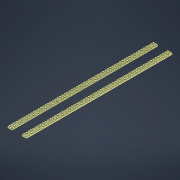
# Autodesk Inventor part: 110033226_ipt_39_背流基座
Saved by Autodesk Inventor 2022 (Build 260153000, 153)
## iProperties
Created: 2022-06-26
Part Number: 110033226_ipt_39_背流基座
Material: 一般
Document SubType Name: Modeling
Designer: User
Density: 1 g/cm^3
Appearance: 預設
Author: User
Autodesk Inventor part; units mm, degrees
ref_plane "YZ Plane" through (0, 0, 0) normal (1, 0, 0) x (0, 1, 0)
ref_plane "XZ Plane" through (0, 0, 0) normal (0, 1, 0) x (-1, 0, 0)
ref_plane "XY Plane" through (0, 0, 0) normal (0, 0, 1) x (1, 0, 0)
sketch "草圖1" plane through (0, 0, 0) normal (0, 1, 0) x (-1, 0, 0)
  line L0 (0, 0) -> (40, 0)
  line L1 (40, 0) -> (40, -305)
  line L2 (40, -305) -> (0, -305)
  line L3 (0, -305) -> (0, 0)
  circle A0 centre (2.5, -2.5) radius 1.7
  line L4 (10, -305) -> (10, 0)
  line L5 (30, -305) -> (30, 0)
  dimension "d0" = 40
  dimension "d1" = 305
  dimension "d2" = 3.4
  dimension "d3" = 2.5
  dimension "d4" = 2.5
  dimension "d45" = 10
  dimension "d46" = 10
  constraints: 12 end point, 4 point on line, 3 perpendicular, 2 parallel, 1 centre point, 1 horizontal
  measures "d0" distance of L1.end L2.end
  measures "d1" distance of L0.end L1.end
  measures "d2" diameter of A0
  measures "d3" distance from line of L3 A0.centre
  measures "d4" distance from line of L0 A0.centre
  measures "d45" distance between parallel lines of L3 L4
  measures "d46" distance between parallel lines of L1 L5
extrude "擠出1" add sketch "草圖1" along normal blind 2.5 contours L0 L4 L2 L3 | L0 L1 L2 L5 | A0
extrude "擠出2" cut sketch "草圖1" along normal blind 1.5 contours A0
sketch "草圖2" plane through (0, 2.5, 0) normal (0, 1, 0) x (1, 0, 0)
  circle A0 centre (-2.5, 2.5) radius 1.7 projected
  point P0 (0, 0)
extrude "擠出3" add sketch "草圖2" along normal blind 1.5
pattern_linear "矩形陣列3" count 61 spacing 5 along (0, 0, -1) count 2 spacing 5 along (-1, 0, 0) of "擠出3", "擠出2"
sketch "草圖3" plane through (0, 2.5, 0) normal (0, 1, 0) x (1, 0, 0)
  circle A0 centre (-2.5, 2.5) radius 1.7 projected
  line L0 (0, 305) -> (0, 0) projected
  line L1 (-30, 0) -> (-40, 0) projected
  line L2 (-40, 0) -> (-40, 305) projected
  line L3 (-40, 305) -> (-30, 305) projected
  circle A1 centre (-2.5, 7.5) radius 1.7 projected
  circle A2 centre (-2.5, 12.5) radius 1.7 projected
  circle A3 centre (-2.5, 17.5) radius 1.7 projected
  circle A4 centre (-2.5, 22.5) radius 1.7 projected
  circle A5 centre (-2.5, 27.5) radius 1.7 projected
  circle A6 centre (-2.5, 32.5) radius 1.7 projected
  circle A7 centre (-2.5, 37.5) radius 1.7 projected
  circle A8 centre (-2.5, 42.5) radius 1.7 projected
  circle A9 centre (-2.5, 47.5) radius 1.7 projected
  circle A10 centre (-2.5, 52.5) radius 1.7 projected
  circle A11 centre (-2.5, 57.5) radius 1.7 projected
  circle A12 centre (-2.5, 62.5) radius 1.7 projected
  circle A13 centre (-2.5, 67.5) radius 1.7 projected
  circle A14 centre (-2.5, 72.5) radius 1.7 projected
  circle A15 centre (-2.5, 77.5) radius 1.7 projected
  circle A16 centre (-2.5, 82.5) radius 1.7 projected
  circle A17 centre (-2.5, 87.5) radius 1.7 projected
  circle A18 centre (-2.5, 92.5) radius 1.7 projected
  circle A19 centre (-2.5, 97.5) radius 1.7 projected
  circle A20 centre (-2.5, 102.5) radius 1.7 projected
  circle A21 centre (-2.5, 107.5) radius 1.7 projected
  circle A22 centre (-2.5, 112.5) radius 1.7 projected
  circle A23 centre (-2.5, 117.5) radius 1.7 projected
  circle A24 centre (-2.5, 122.5) radius 1.7 projected
  circle A25 centre (-2.5, 127.5) radius 1.7 projected
  circle A26 centre (-2.5, 132.5) radius 1.7 projected
  circle A27 centre (-2.5, 137.5) radius 1.7 projected
  circle A28 centre (-2.5, 142.5) radius 1.7 projected
  circle A29 centre (-2.5, 147.5) radius 1.7 projected
  circle A30 centre (-2.5, 152.5) radius 1.7 projected
  circle A31 centre (-2.5, 157.5) radius 1.7 projected
  circle A32 centre (-2.5, 162.5) radius 1.7 projected
  circle A33 centre (-2.5, 167.5) radius 1.7 projected
  circle A34 centre (-2.5, 172.5) radius 1.7 projected
  circle A35 centre (-2.5, 177.5) radius 1.7 projected
  circle A36 centre (-2.5, 182.5) radius 1.7 projected
  circle A37 centre (-2.5, 187.5) radius 1.7 projected
  circle A38 centre (-2.5, 192.5) radius 1.7 projected
  circle A39 centre (-2.5, 197.5) radius 1.7 projected
  circle A40 centre (-2.5, 202.5) radius 1.7 projected
  circle A41 centre (-2.5, 207.5) radius 1.7 projected
  circle A42 centre (-2.5, 212.5) radius 1.7 projected
  circle A43 centre (-2.5, 217.5) radius 1.7 projected
  circle A44 centre (-2.5, 222.5) radius 1.7 projected
  circle A45 centre (-2.5, 227.5) radius 1.7 projected
  circle A46 centre (-2.5, 232.5) radius 1.7 projected
  circle A47 centre (-2.5, 237.5) radius 1.7 projected
  circle A48 centre (-2.5, 242.5) radius 1.7 projected
  circle A49 centre (-2.5, 247.5) radius 1.7 projected
  circle A50 centre (-2.5, 252.5) radius 1.7 projected
  circle A51 centre (-2.5, 257.5) radius 1.7 projected
  circle A52 centre (-2.5, 262.5) radius 1.7 projected
  circle A53 centre (-2.5, 267.5) radius 1.7 projected
  circle A54 centre (-2.5, 272.5) radius 1.7 projected
  circle A55 centre (-2.5, 277.5) radius 1.7 projected
  circle A56 centre (-2.5, 282.5) radius 1.7 projected
  circle A57 centre (-2.5, 287.5) radius 1.7 projected
  circle A58 centre (-2.5, 292.5) radius 1.7 projected
  circle A59 centre (-2.5, 297.5) radius 1.7 projected
  circle A60 centre (-2.5, 302.5) radius 1.7 projected
  circle A61 centre (-7.5, 2.5) radius 1.7 projected
  circle A62 centre (-7.5, 7.5) radius 1.7 projected
  circle A63 centre (-7.5, 12.5) radius 1.7 projected
  circle A64 centre (-7.5, 17.5) radius 1.7 projected
  circle A65 centre (-7.5, 22.5) radius 1.7 projected
  circle A66 centre (-7.5, 27.5) radius 1.7 projected
  circle A67 centre (-7.5, 32.5) radius 1.7 projected
  circle A68 centre (-7.5, 37.5) radius 1.7 projected
  circle A69 centre (-7.5, 42.5) radius 1.7 projected
  circle A70 centre (-7.5, 47.5) radius 1.7 projected
  circle A71 centre (-7.5, 52.5) radius 1.7 projected
  circle A72 centre (-7.5, 57.5) radius 1.7 projected
  circle A73 centre (-7.5, 62.5) radius 1.7 projected
  circle A74 centre (-7.5, 67.5) radius 1.7 projected
  circle A75 centre (-7.5, 72.5) radius 1.7 projected
  circle A76 centre (-7.5, 77.5) radius 1.7 projected
  circle A77 centre (-7.5, 82.5) radius 1.7 projected
  circle A78 centre (-7.5, 87.5) radius 1.7 projected
  circle A79 centre (-7.5, 92.5) radius 1.7 projected
  circle A80 centre (-7.5, 97.5) radius 1.7 projected
  circle A81 centre (-7.5, 102.5) radius 1.7 projected
  circle A82 centre (-7.5, 107.5) radius 1.7 projected
  circle A83 centre (-7.5, 112.5) radius 1.7 projected
  circle A84 centre (-7.5, 117.5) radius 1.7 projected
  circle A85 centre (-7.5, 122.5) radius 1.7 projected
  circle A86 centre (-7.5, 127.5) radius 1.7 projected
  circle A87 centre (-7.5, 132.5) radius 1.7 projected
  circle A88 centre (-7.5, 137.5) radius 1.7 projected
  circle A89 centre (-7.5, 142.5) radius 1.7 projected
  circle A90 centre (-7.5, 147.5) radius 1.7 projected
  circle A91 centre (-7.5, 152.5) radius 1.7 projected
  circle A92 centre (-7.5, 157.5) radius 1.7 projected
  circle A93 centre (-7.5, 162.5) radius 1.7 projected
  circle A94 centre (-7.5, 167.5) radius 1.7 projected
  circle A95 centre (-7.5, 172.5) radius 1.7 projected
  circle A96 centre (-7.5, 177.5) radius 1.7 projected
  circle A97 centre (-7.5, 182.5) radius 1.7 projected
  circle A98 centre (-7.5, 187.5) radius 1.7 projected
  circle A99 centre (-7.5, 192.5) radius 1.7 projected
  circle A100 centre (-7.5, 197.5) radius 1.7 projected
  circle A101 centre (-7.5, 202.5) radius 1.7 projected
  circle A102 centre (-7.5, 207.5) radius 1.7 projected
  circle A103 centre (-7.5, 212.5) radius 1.7 projected
  circle A104 centre (-7.5, 217.5) radius 1.7 projected
  circle A105 centre (-7.5, 222.5) radius 1.7 projected
  circle A106 centre (-7.5, 227.5) radius 1.7 projected
  circle A107 centre (-7.5, 232.5) radius 1.7 projected
  circle A108 centre (-7.5, 237.5) radius 1.7 projected
  circle A109 centre (-7.5, 242.5) radius 1.7 projected
  circle A110 centre (-7.5, 247.5) radius 1.7 projected
  circle A111 centre (-7.5, 252.5) radius 1.7 projected
  circle A112 centre (-7.5, 257.5) radius 1.7 projected
  circle A113 centre (-7.5, 262.5) radius 1.7 projected
  circle A114 centre (-7.5, 267.5) radius 1.7 projected
  circle A115 centre (-7.5, 272.5) radius 1.7 projected
  circle A116 centre (-7.5, 277.5) radius 1.7 projected
  circle A117 centre (-7.5, 282.5) radius 1.7 projected
  circle A118 centre (-7.5, 287.5) radius 1.7 projected
  circle A119 centre (-7.5, 292.5) radius 1.7 projected
  circle A120 centre (-7.5, 297.5) radius 1.7 projected
  circle A121 centre (-7.5, 302.5) radius 1.7 projected
  circle A122 centre (-37.5, 2.5) radius 1.7
  line L4 (-30, 305) -> (-30, 0) projected
  line L5 (0, 0) -> (-10, 0) projected
  line L6 (-10, 0) -> (-10, 305) projected
  line L7 (-10, 305) -> (0, 305) projected
  dimension "d26" = 3.4
  dimension "d27" = 2.5
  dimension "d28" = 2.5
  constraints: 1 centre point
  measures "d26" diameter of A122
  measures "d27" distance from line of L2 A122.centre
  measures "d28" distance from line of L1 A122.centre
extrude "擠出4" add sketch "草圖3" along normal blind 1.5 contours A122
pattern_linear "矩形陣列4" count 61 spacing 5 along (0, 0, -1) count 2 spacing 5 along (1, 0, 0) of "擠出4"
sketch "草圖4" plane through (0, 0, 0) normal (0, -1, 0) x (1, 0, 0)
  circle A0 centre (-37.5, -2.5) radius 1.7 projected
  point P0 (0, 0)
extrude "擠出5" cut sketch "草圖4" against normal blind 1.5
pattern_linear "矩形陣列5" count 2 spacing 5 along (1, 0, 0) count 61 spacing 5 along (0, 0, -1) of "擠出5"
